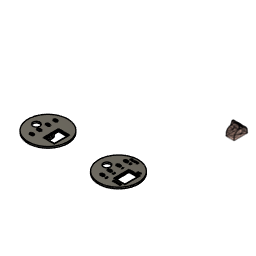
Flap Switch V1 (Autodesk Fusion 360 design; units mm, degrees)
Autodesk Fusion 360 part; units mm, degrees
sketch "Sketch1" plane through (0, 0, 0) normal (0, 0, 1) x (1, 0, 0)
  circle A0 centre (-11, -1) radius 28
  circle A1 centre (-26.8314, -1.5679) radius 5
  line L0 (-19.0596, -5) -> (-16.7152, -5)
  line L1 (-19.3936, -7.9) -> (-16.4275, -7.9)
  arc A2 (-16.4275, -7.9) -> (-16.7152, -5) centre (-16.7152, -6.4643) ccw
  arc A3 (-19.0596, -5) -> (-19.3936, -7.9) centre (-19.0596, -6.4692) ccw
  line L2 (-19.3936, -7.9) -> (-16.4275, -7.9)
  arc A4 (-19.0596, -5) -> (-19.3936, -7.9) centre (-19.0596, -6.4692) ccw
  circle A5 centre (-26.8314, -1.5679) radius 5
  line L3 (-19.0596, -5) -> (-16.7152, -5)
  arc A6 (-16.4275, -7.9) -> (-16.7152, -5) centre (-16.7152, -6.4643) ccw
  line L4 (-19.0596, 7.5) -> (-16.7152, 7.5)
  arc A7 (-19.0596, 7.5) -> (-19.3936, 4.6) centre (-19.0596, 6.0308) ccw
  line L5 (-19.3936, 4.6) -> (-16.4275, 4.6)
  arc A8 (-16.4275, 4.6) -> (-16.7152, 7.5) centre (-16.7152, 6.0357) ccw
  arc A9 (-16.4275, 15.1) -> (-16.7152, 18) centre (-16.7152, 16.5357) ccw
  line L6 (-19.0596, 18) -> (-16.7152, 18)
  arc A10 (-19.0596, 18) -> (-19.3936, 15.1) centre (-19.0596, 16.5308) ccw
  line L7 (-19.3936, 15.1) -> (-16.4275, 15.1)
  line L8 (-19.3936, -18.4) -> (-16.4275, -18.4)
  arc A11 (-16.4275, -18.4) -> (-16.7152, -15.5) centre (-16.7152, -16.9643) ccw
  line L9 (-19.0596, -15.5) -> (-16.7152, -15.5)
  arc A12 (-19.0596, -15.5) -> (-19.3936, -18.4) centre (-19.0596, -16.9692) ccw
  line L10 (8.5, 7) -> (-4, 7)
  line L11 (-4, 7) -> (-4, -11.5)
  line L12 (-4, -11.5) -> (8.5, -11.5)
  line L13 (8.5, -11.5) -> (8.5, 7)
  line L14 (10, 8.5) -> (-5.5, 8.5)
  line L15 (-5.5, 8.5) -> (-5.5, -13)
  line L16 (-5.5, -13) -> (10, -13)
  line L17 (10, -13) -> (10, 8.5)
  dimension "d1" = 56
  dimension "d2" = 10
  dimension "d3" = 10
  dimension "d4" = 12.5
  dimension "d5" = 18.5
  dimension "d6" = 1.5
  constraint horizontal L0
  constraint parallel L0 L1
  constraint tangent L0 A2
  constraint tangent L0 A3
  constraint horizontal L3
  constraint parallel L2 L3
  constraint tangent L3 A6
  constraint tangent A4 L3
  constraint horizontal L4
  constraint parallel L4 L5
  constraint horizontal L6
  constraint parallel L6 L7
  constraint horizontal L9
  constraint tangent A11 L9
  constraint tangent L9 A12
  constraint horizontal L10
  constraint vertical L11
  constraint horizontal L12
  constraint vertical L13
  measures "d1" diameter of A0
  measures "d2" diameter of A1
  measures "d3" diameter of A5
  measures "d4" distance of L10.start L10.end
  measures "d5" distance of L10.start L12.end
extrude "Extrude1" add sketch "Sketch1" along normal blind 2 contours L14 L15 L16 L17 makes body 1
extrude "Extrude2" add sketch "Sketch1" against normal blind 2 separate body contours A0 | L14 L15 L16 L17 makes body 2
fillet "Fillet1" radius 0.5 16 edges at (-20.5192, 6.1989, 0) (-17.8874, 7.5, 0) (-15.2581, 6.1803, 0) (-17.9106, 4.6, 0) (-17.9106, 15.1, 0) (-20.5192, 16.6989, 0) (-17.8874, 18, 0) (-15.2581, 16.6803, 0) (-20.5192, -6.3011, 0) (-17.8874, -5, 0) (-15.2581, -6.3197, 0) (-17.9106, -7.9, 0) (-20.5192, -16.8011, 0) (-17.8874, -15.5, 0) (-15.2581, -16.8197, 0) (-17.9106, -18.4, 0) on bodies 2
extrude "Extrude3" cut 1 faces at (-5, -5.3333, 0) along direction (0, 0, -1) blind 1 on bodies 1 bodies 2
move_face "OffsetFaces1" offset -0.05 4 faces at (-0.3333, -13, -0.3333) (-5.5, 1.3333, -0.3333) (4.8333, 8.5, -0.3333) (10, -5.8333, -0.3333) on bodies 2
move_body "Move1" bodies 1 to x (1, 0, 0) y (0, 1, 0) z (0, 0, 1) at (0, 0, -1)
copy_body "Body->Comp1" bodies 2 removing the originals makes body 3 in component "Face Plate"
copy_body "Body->Comp2" bodies 1 removing the originals makes body 4 in component "Connector Bar"
copy_body "CopyPasteBodies1" bodies 3 makes body 5 in component "Face Plate"
move_body "Move1'" bodies 5 to x (1, 0, 0) y (0, 1, 0) z (0, 0, 1) at (100, 0, 0) in component "Face Plate"
sketch "Sketch1 (2)" plane through (0, 0, 0) normal (0, 0, 1) x (-1, 0, 0) in component "Face Plate"
  line L0 (-94.45, -8.55) -> (-110.05, -8.55)
  line L1 (-110.05, -8.55) -> (-110.05, 13.05)
  line L2 (-110.05, 13.05) -> (-94.45, 13.05)
  line L3 (-94.45, 13.05) -> (-94.45, -8.55)
  arc A0 (-80.9404, 4.5) -> (-80.553, 8.4) centre (-80.9404, 6.4692) ccw
  line L4 (-80.9404, 4.5) -> (-83.2848, 4.5)
  arc A1 (-83.6185, 8.4) -> (-83.2848, 4.5) centre (-83.2848, 6.4643) ccw
  line L5 (-83.6185, 8.4) -> (-80.553, 8.4)
  arc A2 (-80.9404, -8) -> (-80.553, -4.1) centre (-80.9404, -6.0308) ccw
  line L6 (-80.9404, -8) -> (-83.2848, -8)
  arc A3 (-83.6185, -4.1) -> (-83.2848, -8) centre (-83.2848, -6.0357) ccw
  line L7 (-83.6185, -4.1) -> (-80.553, -4.1)
  circle A4 centre (-73.1686, 1.5679) radius 5
  circle A5 centre (-89, 1) radius 28
  arc A6 (-80.9404, -18.5) -> (-80.553, -14.6) centre (-80.9404, -16.5308) ccw
  line L8 (-80.9404, -18.5) -> (-83.2848, -18.5)
  arc A7 (-83.6185, -14.6) -> (-83.2848, -18.5) centre (-83.2848, -16.5357) ccw
  line L9 (-83.6185, -14.6) -> (-80.553, -14.6)
  arc A8 (-80.9404, 15) -> (-80.553, 18.9) centre (-80.9404, 16.9692) ccw
  line L10 (-80.9404, 15) -> (-83.2848, 15)
  arc A9 (-83.6185, 18.9) -> (-83.2848, 15) centre (-83.2848, 16.9643) ccw
  line L11 (-83.6185, 18.9) -> (-80.553, 18.9)
  line L12 (-82.9418, -21.0777) -> (-93.258, -21.0917) construction
  line L13 (-93.258, -21.0917) -> (-93.2545, -23.6422) construction
  line L14 (-93.2545, -23.6422) -> (-82.9384, -23.6282) construction
  line L15 (-82.9384, -23.6282) -> (-82.9418, -21.0777) construction
  line L16 (-87.3683, -15.602) -> (-89.7047, -15.6052) construction
  line L17 (-89.7047, -15.6052) -> (-89.7012, -18.1557) construction
  line L18 (-89.7012, -18.1557) -> (-87.3648, -18.1525) construction
  line L19 (-87.3648, -18.1525) -> (-87.3683, -15.602) construction
  line L20 (-87.3683, -4.602) -> (-89.7047, -4.6052) construction
  line L21 (-89.7047, -4.6052) -> (-89.7012, -7.1557) construction
  line L22 (-89.7012, -7.1557) -> (-87.3648, -7.1525) construction
  line L23 (-87.3648, -7.1525) -> (-87.3683, -4.602) construction
  line L24 (-87.3683, 7.898) -> (-89.7047, 7.8948) construction
  line L25 (-89.7047, 7.8948) -> (-89.7012, 5.3443) construction
  line L26 (-89.7012, 5.3443) -> (-87.3648, 5.3475) construction
  line L27 (-87.3648, 5.3475) -> (-87.3683, 7.898) construction
  line L28 (-87.3683, 18.398) -> (-89.7047, 18.3948) construction
  line L29 (-89.7047, 18.3948) -> (-89.7012, 15.8443) construction
  line L30 (-89.7012, 15.8443) -> (-87.3648, 15.8475) construction
  line L31 (-87.3648, 15.8475) -> (-87.3683, 18.398) construction
  line L32 (-96.9285, 17.4515) -> (-99.265, 17.4483) construction
  line L33 (-99.265, 17.4483) -> (-99.2615, 14.8978) construction
  line L34 (-99.2615, 14.8978) -> (-96.925, 14.901) construction
  line L35 (-96.925, 14.901) -> (-96.9285, 17.4515) construction
  line L36 (-103.742, -10.0003) -> (-106.0784, -10.0035) construction
  line L37 (-106.0784, -10.0035) -> (-106.0749, -12.554) construction
  line L38 (-106.0749, -12.554) -> (-103.7385, -12.5508) construction
  line L39 (-103.7385, -12.5508) -> (-103.742, -10.0003) construction
  dimension "d16" = 2.5
  dimension "d17" = 3
  dimension "d18" = 3
  dimension "d19" = 3
  dimension "d20" = 3
  dimension "d21" = 2.5
  dimension "d22" = 2.5
  text T0 "FLAPS" font "Arial" height 2.5 align left top in box 10.3161 x 2.5504 at (-82.9418, -21.0777) x (-0.999999, -0.001358) y (0.001358, -0.999999) spacing 1 kerned
  text T1 "0" font "Arial" height 3 align left top in box 2.3364 x 2.5505 at (-87.3683, -15.602) x (-0.999999, -0.001369) y (0.001369, -0.999999) spacing 1 kerned
  text T2 "1" font "Arial" height 3 align left top in box 2.3364 x 2.5505 at (-87.3683, -4.602) x (-0.999999, -0.001369) y (0.001369, -0.999999) spacing 1 kerned
  text T3 "2" font "Arial" height 3 align left top in box 2.3364 x 2.5505 at (-87.3683, 7.898) x (-0.999999, -0.001369) y (0.001369, -0.999999) spacing 1 kerned
  text T4 "3" font "Arial" height 3 align left top in box 2.3364 x 2.5505 at (-87.3683, 18.398) x (-0.999999, -0.001369) y (0.001369, -0.999999) spacing 1 kerned
  text T5 "DOWN" font "Arial" height 2.5 align left top in box 2.3364 x 2.5505 at (-96.9285, 17.4515) x (-0.999999, -0.001369) y (0.001369, -0.999999) spacing 1 kerned
  text T6 "UP" font "Arial" height 2.5 align left top in box 2.3364 x 2.5505 at (-103.742, -10.0003) x (-0.999999, -0.001369) y (0.001369, -0.999999) spacing 1 kerned
extrude "Extrude1'" cut sketch "Sketch1 (2)" against normal blind 0.5 text T4 T3 T6 T2 T1 T0 T5 bodies 5 in component "Face Plate"
sketch "Sketch2" plane through (0, 0, -2) normal (0, 0, -1) x (1, 0, 0)
  arc A0 (-19.3936, 7.9) -> (-19.0596, 5) centre (-19.0596, 6.4692) ccw
  line L0 (-19.3936, 7.9) -> (-16.4275, 7.9)
  arc A1 (-16.7152, 5) -> (-16.4275, 7.9) centre (-16.7152, 6.4643) ccw
  line L1 (-16.7152, 5) -> (-19.0596, 5)
  circle A2 centre (-26.8314, 1.5679) radius 5
  arc A3 (-19.3936, -4.6) -> (-19.0596, -7.5) centre (-19.0596, -6.0308) ccw
  line L2 (-19.3936, -4.6) -> (-16.4275, -4.6)
  arc A4 (-16.7152, -7.5) -> (-16.4275, -4.6) centre (-16.7152, -6.0357) ccw
  line L3 (-16.7152, -7.5) -> (-19.0596, -7.5)
  line L4 (8.5, 11.5) -> (8.5, -7)
  line L5 (8.5, -7) -> (-4, -7)
  line L6 (-4, -7) -> (-4, 11.5)
  line L7 (-4, 11.5) -> (8.5, 11.5)
  arc A5 (-19.3936, -15.1) -> (-19.0596, -18) centre (-19.0596, -16.5308) ccw
  line L8 (-19.3936, -15.1) -> (-16.4275, -15.1)
  arc A6 (-16.7152, -18) -> (-16.4275, -15.1) centre (-16.7152, -16.5357) ccw
  line L9 (-16.7152, -18) -> (-19.0596, -18)
  arc A7 (-19.3936, 18.4) -> (-19.0596, 15.5) centre (-19.0596, 16.9692) ccw
  line L10 (-19.3936, 18.4) -> (-16.4275, 18.4)
  arc A8 (-16.7152, 15.5) -> (-16.4275, 18.4) centre (-16.7152, 16.9643) ccw
  line L11 (-16.7152, 15.5) -> (-19.0596, 15.5)
  circle A9 centre (-11, 1) radius 28
  line L12 (-16.7152, -17.9) -> (-19.0596, -17.9)
  arc A10 (-19.3819, -15.2) -> (-19.0596, -17.9) centre (-19.0596, -16.5308) ccw
  line L13 (-19.3819, -15.2) -> (-16.4376, -15.2)
  arc A11 (-16.7152, -17.9) -> (-16.4376, -15.2) centre (-16.7152, -16.5357) ccw
  arc A12 (-19.33, -15.6) -> (-19.0596, -17.5) centre (-19.0596, -16.5308) ccw
  line L14 (-16.7152, -17.5) -> (-19.0596, -17.5)
  arc A13 (-16.7152, -17.5) -> (-16.4823, -15.6) centre (-16.7152, -16.5357) ccw
  line L15 (-19.33, -15.6) -> (-16.4823, -15.6)
  dimension "d25" = 0.1
  dimension "d26" = 0.5
extrude "Extrude4" add sketch "Sketch2" against normal blind 1.25 separate body contours A12 L14 A13 L15 makes body 6
extrude "Extrude5" add sketch "Sketch2" along normal blind -1.25 and the other way blind 0 contours L12 A10 L13 A11 bodies 6
sketch "Sketch3" plane through (0, 0, -2) normal (0, 0, -1) x (1, 0, 0)
  arc A0 (-19.3819, -15.2) -> (-19.0596, -17.9) centre (-19.0596, -16.5308) ccw
  line L0 (-19.0596, -17.9) -> (-16.7152, -17.9)
  arc A1 (-16.7152, -17.9) -> (-16.4376, -15.2) centre (-16.7152, -16.5357) ccw
  line L1 (-16.4376, -15.2) -> (-19.3819, -15.2)
  circle A2 centre (-17.8874, -16.6753) radius 1.1
  dimension "d33" = 2.2
  measures "d33" diameter of A2
extrude "Extrude6" cut sketch "Sketch3" against normal blind 0.6 contours A2 bodies 6
sketch "Sketch4" plane through (0, 0, -2) normal (0, 0, -1) x (1, 0, 0)
  circle A0 centre (-17.8874, -16.6753) radius 1.1
  arc A1 (-19.3819, -15.2) -> (-19.0596, -17.9) centre (-19.0596, -16.5308) ccw
  line L0 (-19.0596, -17.9) -> (-16.7152, -17.9)
  arc A2 (-16.7152, -17.9) -> (-16.4376, -15.2) centre (-16.7152, -16.5357) ccw
  line L1 (-16.4376, -15.2) -> (-19.3819, -15.2)
  line L2 (-20.8874, -14.1753) -> (-14.8874, -14.1753)
  line L3 (-14.8874, -14.1753) -> (-14.8874, -19.1753)
  line L4 (-14.8874, -19.1753) -> (-20.8874, -19.1753)
  line L5 (-20.8874, -19.1753) -> (-20.8874, -14.1753)
  line L6 (-20.8874, -14.1753) -> (-14.8874, -19.1753) construction
  line L7 (-14.8874, -14.1753) -> (-20.8874, -19.1753) construction
  point P0 (-17.8874, -16.6753)
  dimension "d36" = 6
  dimension "d37" = 5
  constraint horizontal L2
  constraint perpendicular L2 L3
  constraint parallel L2 L4
  constraint parallel L3 L5
  constraint coincident L6 P0
  constraint coincident L7 P0
  constraint coincident P0 A0.centre
  measures "d36" distance of L3.end L4.end
  measures "d37" distance of L2.end L3.end
extrude "Extrude7" add sketch "Sketch4" along normal blind 4 contours A1 L0 A2 L1 | L2 L3 L4 L5 bodies 6
sketch "Sketch5" plane through (0, 0, -6) normal (0, 0, -1) x (1, 0, 0)
  circle A0 centre (-17.8874, -16.6753) radius 1.1
  line L0 (-20.8874, -19.1753) -> (-14.8874, -19.1753)
  line L1 (-14.8874, -19.1753) -> (-14.8874, -14.1753)
  line L2 (-14.8874, -14.1753) -> (-20.8874, -14.1753)
  line L3 (-20.8874, -14.1753) -> (-20.8874, -19.1753)
  line L4 (-18.9874, -15.3253) -> (-16.7874, -15.3253)
  line L5 (-16.7874, -15.3253) -> (-16.7874, -18.0253)
  line L6 (-16.7874, -18.0253) -> (-18.9874, -18.0253)
  line L7 (-18.9874, -18.0253) -> (-18.9874, -15.3253)
  line L8 (-18.9874, -15.3253) -> (-16.7874, -18.0253) construction
  line L9 (-16.7874, -15.3253) -> (-18.9874, -18.0253) construction
  point P0 (-17.8874, -16.6753)
  dimension "d40" = 2.2
  dimension "d41" = 2.7
  constraint horizontal L4
  constraint perpendicular L4 L5
  constraint parallel L4 L6
  constraint parallel L5 L7
  constraint coincident L8 P0
  constraint coincident L9 P0
  constraint coincident P0 A0.centre
  measures "d40" distance of L5.end L6.end
  measures "d41" distance of L4.end L5.end
extrude "Extrude8" add sketch "Sketch5" along normal blind 1.5 bodies 6
fillet "Fillet2" radius 2.5 4 edges at (-14.8874, 14.1753, -4.75) (-14.8874, 19.1753, -4.75) (-20.8874, 19.1753, -4.75) (-20.8874, 14.1753, -4.75) on bodies 6
copy_body "Body->Comp3" bodies 6 removing the originals makes body 7 in component "LED Holders"
copy_body "CopyPasteBodies1'" bodies 7 makes body 8
move_body "Move2" bodies 8 to x (1, 0, 0) y (0, 1, 0) z (0, 0, 1) at (0, -10.5, 0)
copy_body "CutPasteBodies1" bodies 8 removing the originals makes body 9 in component "LED Holders"
copy_body "CopyPasteBodies2" bodies 7 9 makes body 10 makes body 11
move_body "Move3" bodies 10 11 to x (1, 0, 0) y (0, 1, 0) z (0, 0, 1) at (0, -23, 0)
copy_body "CutPasteBodies2" bodies 10 11 removing the originals makes body 12 makes body 13 in component "LED Holders"
other "Base Mesh Feature2"
sketch "Sketch6" plane through (0, 0, 0) normal (1, 0, 0) x (0, 1, 0)
  line L0 (118.3669, 3.6902) -> (118.6562, 5.3488)
  line L1 (118.8118, 5.8291) -> (119.4016, 7.0374)
  line L2 (119.7044, 7.4772) -> (120.6533, 8.4922)
  line L3 (121.035, 8.8021) -> (122.2863, 9.5607)
  line L4 (122.631, 9.7226) -> (124.3, 10.3)
  arc A0 (124.3, 10.3) -> (125.3, 11.3) centre (123.7711, 11.8289) ccw
  line L5 (125.3, 11.3) -> (126.07, 13.88)
  arc A1 (126.1484, 14.0986) -> (126.07, 13.88) centre (128.1211, 13.2679) ccw
  line L6 (127.8073, 15.2) -> (127.7683, 15.2)
  line L7 (127.7683, 3.6902) -> (127.7683, 15.2)
  arc A2 (118.8118, 5.8291) -> (118.6562, 5.3488) centre (120.4294, 5.0396) ccw
  arc A3 (119.7044, 7.4772) -> (119.4016, 7.0374) centre (121.0192, 6.2479) ccw
  arc A4 (121.035, 8.8021) -> (120.6533, 8.4922) centre (121.9682, 7.2629) ccw
  arc A5 (122.631, 9.7226) -> (122.2863, 9.5607) centre (123.2195, 8.0215) ccw
  arc A6 (127.8073, 15.2) -> (126.1484, 14.0986) centre (127.8073, 13.4) ccw
  line L8 (127.7683, 3.6902) -> (118.3669, 3.6902)
  line L9 (130.2366, 11.3) -> (129.4666, 13.88)
  arc A7 (129.4666, 13.88) -> (129.3882, 14.0986) centre (127.4155, 13.2679) ccw
  line L10 (134.5016, 8.8021) -> (133.2503, 9.5607)
  arc A8 (134.8832, 8.4922) -> (134.5016, 8.8021) centre (133.5684, 7.2629) ccw
  line L11 (136.7247, 5.8291) -> (136.135, 7.0374)
  arc A9 (136.135, 7.0374) -> (135.8322, 7.4772) centre (134.5174, 6.2479) ccw
  arc A10 (129.3882, 14.0986) -> (127.7293, 15.2) centre (127.7293, 13.4) ccw
  line L12 (135.8322, 7.4772) -> (134.8832, 8.4922)
  line L13 (137.1697, 3.6902) -> (136.8804, 5.3488)
  line L14 (132.9056, 9.7226) -> (131.2366, 10.3)
  arc A11 (136.8804, 5.3488) -> (136.7247, 5.8291) centre (135.1071, 5.0396) ccw
  line L15 (127.7683, 3.6902) -> (137.1697, 3.6902)
  arc A12 (130.2366, 11.3) -> (131.2366, 10.3) centre (131.7655, 11.8289) ccw
  arc A13 (133.2503, 9.5607) -> (132.9056, 9.7226) centre (132.3171, 8.0215) ccw
  dimension "d46" = 1.8
  constraint tangent L4 A0
  constraint tangent L5 A1
  constraint horizontal L6
  constraint coincident L6 L7.end
  constraint perpendicular L6 L7
  constraint tangent L0 A2
  constraint tangent L1 A2
  constraint tangent L1 A3
  constraint tangent L2 A3
  constraint equal A2 A3
  constraint tangent L2 A4
  constraint tangent L3 A4
  constraint equal A2 A4
  constraint tangent L3 A5
  constraint tangent L4 A5
  constraint equal A2 A5
  constraint tangent A1 A6
  constraint tangent L6 A6
  constraint equal A2 A6
  constraint symmetric L0.start L7 L13.start
  constraint symmetric L4.end L7 L14.end
  constraint symmetric A0.end L7 L9.start
  constraint symmetric A0 L7 A12
  constraint symmetric L5.end L7 L9.end
  constraint symmetric A1 L7 A7
  constraint symmetric L8.start L7 L15.start
  constraint symmetric L7 L0.end L13.end
  constraint symmetric L7 L1.start L11.start
  constraint symmetric L7 A2 A11
  constraint symmetric L7 L1.end L11.end
  constraint symmetric L7 L2.start A9.end
  constraint symmetric L7 A3 A9
  constraint symmetric L7 L2.end A8.start
  constraint symmetric L7 L3.start L10.start
  constraint symmetric L7 A4 A8
  constraint symmetric L7 L3.end L10.end
  constraint symmetric L7 L4.start L14.start
  constraint symmetric L7 A5 A13
  constraint symmetric L7 L6.start A10.end
  constraint symmetric L7 A1.start A7.end
  constraint symmetric L7 A6 A10
  measures "d46" radius of A2
extrude "Extrude9" add sketch "Sketch6" along normal blind 11.3 separate body makes body 14
move_body "Move4" bodies 14 to x (1, 0, 0) y (0, 1, 0) z (0, 0, 1) at (-3.4, -130, -5.69)
scale "Scale1" factors (1, 0.95, 1) about (7.9, -4.7, 5.61) bodies 14
copy_body "Body->Comp4" bodies 14 removing the originals makes body 15 in component "Flap Switch"
sketch "Sketch1 (3)" plane through (-3.4, 0, 0) normal (-1, 0, 0) x (0, -1, 0) in component "Flap Switch"
  line L0 (-6.5762, -1.9998) -> (11.2865, -1.9998)
  line L1 (11.2865, -1.9998) -> (11.0116, -0.3412)
  ellipse E0 centre (9.3271, -0.6504) end of major axis (9.3271, -2.4504) minor radius 1.71 (11.0116, -0.3412) -> (10.8638, 0.1391) ccw
  line L2 (10.8638, 0.1391) -> (10.3035, 1.3474)
  ellipse E1 centre (8.7668, 0.5579) end of major axis (8.7668, -1.2421) minor radius 1.71 (10.3035, 1.3474) -> (10.0159, 1.7872) ccw
  line L3 (10.0159, 1.7872) -> (9.1143, 2.8022)
  ellipse E2 centre (7.8652, 1.5729) end of major axis (7.8652, -0.2271) minor radius 1.71 (9.1143, 2.8022) -> (8.7518, 3.1121) ccw
  line L4 (8.7518, 3.1121) -> (7.5631, 3.8707)
  ellipse E3 centre (6.6765, 2.3315) end of major axis (6.6765, 0.5315) minor radius 1.71 (7.5631, 3.8707) -> (7.2356, 4.0326) ccw
  line L5 (7.2356, 4.0326) -> (5.65, 4.61)
  ellipse E4 centre (6.1525, 6.1389) end of major axis (6.1525, 7.7568) minor radius 1.5369 (4.7, 5.61) -> (5.65, 4.61) ccw
  line L6 (4.7, 5.61) -> (3.9685, 8.19)
  ellipse E5 centre (2.02, 7.5779) end of major axis (2.02, 5.4374) minor radius 2.0334 (3.9685, 8.19) -> (3.894, 8.4086) ccw
  ellipse E6 centre (2.3181, 7.71) end of major axis (2.3181, 9.51) minor radius 1.71 (3.894, 8.4086) -> (2.3551, 9.5096) ccw
  ellipse E7 centre (2.3922, 7.71) end of major axis (2.3922, 9.51) minor radius 1.71 (2.3551, 9.5096) -> (0.8163, 8.4086) ccw
  ellipse E8 centre (2.6903, 7.5779) end of major axis (2.6903, 9.7183) minor radius 2.0334 (0.8163, 8.4086) -> (0.7418, 8.19) ccw
  line L7 (0.7418, 8.19) -> (0.0103, 5.61)
  ellipse E9 centre (-1.4422, 6.1389) end of major axis (-1.4422, 4.5211) minor radius 1.5369 (-0.9397, 4.61) -> (0.0103, 5.61) ccw
  line L8 (-0.9397, 4.61) -> (-2.5253, 4.0326)
  ellipse E10 centre (-1.9662, 2.3315) end of major axis (-1.9662, 4.1315) minor radius 1.71 (-2.5253, 4.0326) -> (-2.8528, 3.8707) ccw
  line L9 (-2.8528, 3.8707) -> (-4.0415, 3.1121)
  ellipse E11 centre (-3.155, 1.5729) end of major axis (-3.155, 3.3729) minor radius 1.71 (-4.0415, 3.1121) -> (-4.4041, 2.8022) ccw
  line L10 (-4.4041, 2.8022) -> (-5.3056, 1.7872)
  ellipse E12 centre (-4.0565, 0.5579) end of major axis (-4.0565, 2.3579) minor radius 1.71 (-5.3056, 1.7872) -> (-5.5932, 1.3474) ccw
  line L11 (-5.5932, 1.3474) -> (-6.1535, 0.1391)
  ellipse E13 centre (-4.6168, -0.6504) end of major axis (-4.6168, 1.1496) minor radius 1.71 (-6.1535, 0.1391) -> (-6.3014, -0.3412) ccw
  line L12 (-6.3014, -0.3412) -> (-6.5762, -1.9998)
  line L13 (-6.5762, -1.9998) -> (-1.5762, -1.9998) construction
  line L14 (11.2865, -1.9998) -> (16.2865, -1.9998) construction
  line L15 (-6.5762, -1.9998) -> (-0.5762, -1.9998) construction
  line L16 (11.2865, -1.9998) -> (17.2865, -1.9998) construction
  line L17 (-6.5762, -1.9998) -> (-4.1821, -8.5776)
  line L18 (-6.5762, -1.9998) -> (0.4238, -1.9998) construction
  line L19 (11.2865, -1.9998) -> (8.8923, -8.5776)
  line L20 (11.2865, -1.9998) -> (18.2865, -1.9998) construction
  line L21 (8.8923, -8.5776) -> (-4.1821, -8.5776)
  circle A0 centre (2.3551, -3.2554) radius 1
  dimension "d77" = 70
  dimension "d78" = 7
  dimension "d79" = 110
  dimension "d80" = 7
  dimension "d81" = 2
  constraint horizontal L13
  constraint coincident L0.start L12.end
  constraint horizontal L14
  constraint coincident L0.end L1.start
  constraint horizontal L15
  constraint horizontal L16
  constraint horizontal L18
  constraint horizontal L20
  measures "d77" angle of L17 L18
  measures "d78" distance of L0.start L17.end
  measures "d79" angle of L19 L20
  measures "d80" distance of L0.end L19.end
  measures "d81" diameter of A0
extrude "Extrude1''" add sketch "Sketch1 (3)" against normal blind 11.3 contours L0 L1 E0 L2 E1 L3 E2 L4 E3 L5 E4 L6 E5 E6 E7 E8 L7 E9 L8 E10 L9 E11 L10 E12 L11 E13 L12 bodies 15 in component "Flap Switch"
extrude "Extrude2'" add sketch "Sketch1 (3)" against normal blind 11.3 bodies 15 in component "Flap Switch"
fillet "Fillet3" radius 4.75 2 edges at (2.25, 6.5762, -1.9998) (2.25, -11.2865, -1.9998) on bodies 15 in component "Flap Switch"
sketch "Sketch3 (2)" plane through (0, 0, -8.5776) normal (0, 0, -1) x (1, 0, 0) in component "Flap Switch"
  line L0 (-3.4, 8.8923) -> (-3.4, -4.1821)
  line L1 (-3.4, -4.1821) -> (7.9, -4.1821)
  line L2 (7.9, -4.1821) -> (7.9, 8.8923)
  line L3 (7.9, 8.8923) -> (-3.4, 8.8923)
  line L4 (7.95, -7.6449) -> (-3.45, -7.6449)
  line L5 (-3.45, -7.6449) -> (-3.45, 12.3551)
  line L6 (-3.45, 12.3551) -> (7.95, 12.3551)
  line L7 (7.95, 12.3551) -> (7.95, -7.6449)
  line L8 (7.95, -7.6449) -> (-3.45, 12.3551) construction
  line L9 (-3.45, -7.6449) -> (7.95, 12.3551) construction
  point P0 (2.25, 2.3551)
  dimension "d84" = 11.4
  dimension "d85" = 20
  constraint horizontal L4
  constraint perpendicular L4 L5
  constraint parallel L4 L6
  constraint parallel L5 L7
  constraint coincident L8 P0
  constraint coincident L9 P0
  measures "d84" distance of L5.end L6.end
  measures "d85" distance of L4.end L5.end
extrude "Extrude5'" add 1 faces at (0.3667, -4.5342, -8.5776) along direction (0, 0, -1) blind 2 on bodies 15 bodies 15 in component "Flap Switch"
extrude "Extrude4'" add sketch "Sketch3 (2)" along normal blind 4.5 and the other way blind -2 contours L0 L1 L2 L3 | L4 L5 L6 L7 bodies 15 in component "Flap Switch"
fillet "Fillet4" radius 4 2 edges at (2.25, -8.8923, -10.5776) (2.25, 4.1821, -10.5776) on bodies 15 in component "Flap Switch"
fillet "Fillet6" radius 1 2 edges at (2.25, 7.6449, -10.5776) (2.25, -12.3551, -10.5776) on bodies 15 in component "Flap Switch"
fillet "Fillet8" radius 3 2 edges at (2.25, 4.1821, -8.5776) (2.25, -8.8923, -8.5776) on bodies 15 in component "Flap Switch"
sketch "Sketch4 (2)" plane through (-3.45, 0, 0) normal (-1, 0, 0) x (0, -1, 0) in component "Flap Switch"
  arc A0 (12.3551, -11.4763) -> (11.7937, -10.5776) centre (11.3551, -11.4763) ccw
  line L0 (11.7937, -10.5776) -> (-7.0834, -10.5776)
  arc A1 (-7.0834, -10.5776) -> (-7.6449, -11.4763) centre (-6.6449, -11.4763) ccw
  line L1 (-7.6449, -11.4763) -> (-7.6449, -13.0776)
  line L2 (-7.6449, -13.0776) -> (12.3551, -13.0776)
  line L3 (12.3551, -13.0776) -> (12.3551, -11.4763)
  line L4 (12.3551, -13.0776) -> (6.1051, -23.9029)
  line L5 (12.3551, -13.0776) -> (24.8551, -13.0776) construction
  line L6 (12.3551, -13.0776) -> (10.3551, -13.0776)
  line L7 (10.3551, -13.0776) -> (4.6051, -23.0369)
  line L8 (4.6051, -23.0369) -> (6.1051, -23.9029)
  line L9 (-7.6449, -13.0776) -> (-1.3949, -23.9029)
  line L10 (-7.6449, -13.0776) -> (4.8551, -13.0776) construction
  line L11 (-7.6449, -13.0776) -> (-5.6449, -13.0776)
  line L12 (-5.6449, -13.0776) -> (0.1051, -23.0369)
  line L13 (-5.6449, -13.0776) -> (5.8551, -13.0776) construction
  line L14 (0.1051, -23.0369) -> (-1.3949, -23.9029)
  dimension "d104" = 120
  dimension "d105" = 12.5
  dimension "d106" = 2
  dimension "d107" = 11.5
  dimension "d108" = 60
  dimension "d109" = 12.5
  dimension "d110" = 2
  dimension "d111" = 60
  dimension "d112" = 11.5
  constraint horizontal L5
  constraint coincident L2.end L3.start
  constraint parallel L2 L6
  constraint parallel L4 L7
  constraint horizontal L10
  constraint coincident L1.end L2.start
  constraint parallel L10 L11
  constraint horizontal L13
  measures "d104" angle of L4 L5
  measures "d105" distance of L2.end L4.end
  measures "d106" distance of L2.end L6.end
  measures "d107" distance of L6.end L7.end
  measures "d108" angle of L9 L10
  measures "d109" distance of L1.end L9.end
  measures "d110" distance of L1.end L11.end
  measures "d111" angle of L12 L13
  measures "d112" distance of L11.end L12.end
extrude "Extrude6'" add sketch "Sketch4 (2)" against normal blind 11.4 contours L2 L4 L6 L7 L8 | L2 L9 L11 L12 L14 bodies 15 in component "Flap Switch"
sketch "Sketch2 (2)" plane through (0, 0, -2) normal (0, 0, -1) x (1, 0, 0) in component "Face Plate"
  arc A0 (-19.3936, 7.9) -> (-19.0596, 5) centre (-19.0596, 6.4692) ccw
  line L0 (-19.3936, 7.9) -> (-16.4275, 7.9)
  arc A1 (-16.7152, 5) -> (-16.4275, 7.9) centre (-16.7152, 6.4643) ccw
  line L1 (-16.7152, 5) -> (-19.0596, 5)
  circle A2 centre (-26.8314, 1.5679) radius 5
  arc A3 (-19.3936, -4.6) -> (-19.0596, -7.5) centre (-19.0596, -6.0308) ccw
  line L2 (-19.3936, -4.6) -> (-16.4275, -4.6)
  arc A4 (-16.7152, -7.5) -> (-16.4275, -4.6) centre (-16.7152, -6.0357) ccw
  line L3 (-16.7152, -7.5) -> (-19.0596, -7.5)
  line L4 (8.5, 11.5) -> (8.5, -7)
  line L5 (8.5, -7) -> (-4, -7)
  line L6 (-4, -7) -> (-4, 11.5)
  line L7 (-4, 11.5) -> (8.5, 11.5)
  arc A5 (-19.3936, -15.1) -> (-19.0596, -18) centre (-19.0596, -16.5308) ccw
  line L8 (-19.3936, -15.1) -> (-16.4275, -15.1)
  arc A6 (-16.7152, -18) -> (-16.4275, -15.1) centre (-16.7152, -16.5357) ccw
  line L9 (-16.7152, -18) -> (-19.0596, -18)
  arc A7 (-19.3936, 18.4) -> (-19.0596, 15.5) centre (-19.0596, 16.9692) ccw
  line L10 (-19.3936, 18.4) -> (-16.4275, 18.4)
  arc A8 (-16.7152, 15.5) -> (-16.4275, 18.4) centre (-16.7152, 16.9643) ccw
  line L11 (-16.7152, 15.5) -> (-19.0596, 15.5)
  circle A9 centre (-11, 1) radius 28
  line L12 (-4, 2.25) -> (-7, 2.25)
  line L13 (-7, 2.25) -> (-7, -0.75)
  line L14 (-7, -0.75) -> (-4, -0.75)
  line L15 (-4, -0.75) -> (-4, 2.25)
  line L16 (-7, 2.25) -> (-4, 2.25)
  line L17 (-4, 2.25) -> (-4, 5.25)
  line L18 (-4, 5.25) -> (-7, 5.25)
  line L19 (-7, 5.25) -> (-7, 2.25)
  line L20 (8.5, 2.25) -> (11.5, 2.25)
  line L21 (11.5, 2.25) -> (11.5, 5.25)
  line L22 (11.5, 5.25) -> (8.5, 5.25)
  line L23 (8.5, 5.25) -> (8.5, 2.25)
  line L24 (8.5, 2.25) -> (11.5, 2.25)
  line L25 (11.5, 2.25) -> (11.5, -0.75)
  line L26 (11.5, -0.75) -> (8.5, -0.75)
  line L27 (8.5, -0.75) -> (8.5, 2.25)
  dimension "d115" = 3
  dimension "d116" = 3
  dimension "d117" = 3
  dimension "d118" = 3
  dimension "d119" = 3
  dimension "d120" = 3
  dimension "d121" = 3
  constraint horizontal L12
  constraint vertical L13
  constraint horizontal L14
  constraint vertical L15
  constraint midpoint L6 L12.start
  constraint horizontal L16
  constraint vertical L17
  constraint horizontal L18
  constraint vertical L19
  constraint horizontal L20
  constraint vertical L21
  constraint horizontal L22
  constraint vertical L23
  constraint midpoint L4 L20.start
  constraint horizontal L24
  constraint vertical L25
  constraint horizontal L26
  constraint vertical L27
  measures "d115" distance of L12.start L12.end
  measures "d116" distance of L12.start L14.end
  measures "d117" distance of L12.end L18.end
  measures "d118" distance of L20.start L20.end
  measures "d119" distance of L20.start L22.end
  measures "d120" distance of L20.start L20.end
  measures "d121" distance of L20.start L26.end
extrude "Extrude2''" add sketch "Sketch2 (2)" along normal blind 4 contours L4 L20 L21 L22 L23 L24 | L4 L20 L24 L25 L26 L27 | L6 L12 L16 L17 L18 L19 | L6 L12 L13 L14 L15 L16 bodies 3 in component "Face Plate"
extrude "Extrude3'" cut sketch "Sketch1 (3)" along normal blind 6.5 and the other way blind 22 contours A0 bodies 3 in component "Face Plate"
component "Face Plate" placed x (1, 0, 0) y (0, 1, 0) z (0, 0, 1) at (0, 0, 0)
component "Connector Bar" placed x (1, 0, 0) y (0, 1, 0) z (0, 0, 1) at (0, 0, 0)
component "LED Holders" placed x (1, 0, 0) y (0, 1, 0) z (0, 0, 1) at (0, 0, 0)
component "Flap Switch" placed x (1, 0, 0) y (0, 1, 0) z (0, 0, 1) at (0, 0, 0)
hidden bodies 15
named bodies: "Face Plate No Text", "Face Plate With Text", "0 (1)"
